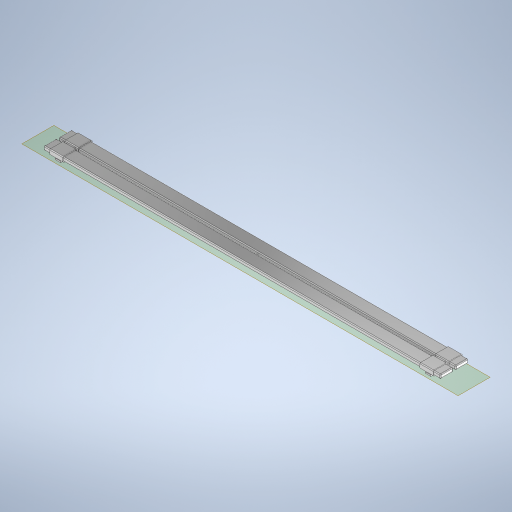
# Autodesk Inventor part: slider
Saved by Autodesk Inventor 2023 (Build 270158000, 158)
## iProperties
Created: 2023-11-22
Part Number: slider
Material: Aluminum 6061
Document SubType Name: Modeling
Designer: Beatrice
Density: 2.7 g/cm^3
Appearance: Chrome - Polished
Author: Beatrice
Autodesk Inventor part; units mm, degrees
ref_plane "YZ Plane" through (0, 0, 0) normal (1, 0, 0) x (0, 1, 0)
sketch "Sketch1" plane through (0, 0, 0) normal (1, 0, 0) x (0, 1, 0)
  line L0 (-1.5, -4.5) -> (-11.85, -4.5) construction
  line L1 (-11.85, -4.5) -> (-11.85, 0.0128) construction
  line L2 (-11.85, 0.0128) -> (0, 0.0128) construction
  line L3 (0, 0.0128) -> (0, 0) construction
  line L4 (0, 0) -> (2, 0) construction
  line L5 (2, 0) -> (2, -26) construction
  line L6 (2, -26) -> (0, -26) construction
  line L7 (0, -26) -> (-11.85, -26) construction
  line L8 (-11.85, -26) -> (-11.85, -21) construction
  line L9 (-11.85, -21) -> (-1.5, -21) construction
  line L10 (-1.5, -21) -> (-1.5, -4.5) construction
  arc A0 (1.25, -12.7436) -> (1.25, -13.2436) centre (1.25, -12.9936) ccw construction
  arc A1 (1.25, -12.7436) -> (1.5, -12.4936) centre (1.25, -12.4936) ccw construction
  line L11 (1.5, -12.4936) -> (1.5, -7.7436) construction
  arc A2 (1.5, -7.7436) -> (1.25, -7.4936) centre (1.25, -7.7436) ccw construction
  line L12 (1.25, -7.4936) -> (-0.25, -7.4936) construction
  arc A3 (-0.25, -7.4936) -> (-0.5, -7.7436) centre (-0.25, -7.7436) ccw construction
  line L13 (-0.5, -7.7436) -> (-0.5, -12.4936) construction
  arc A4 (-0.5, -12.4936) -> (-0.25, -12.7436) centre (-0.25, -12.4936) ccw construction
  arc A5 (-0.25, -13.2436) -> (-0.25, -12.7436) centre (-0.25, -12.9936) ccw construction
  line L14 (-0.25, -13.2436) -> (-0.5, -13.2436) construction
  line L15 (-0.5, -13.2436) -> (-0.5, -18.2436) construction
  arc A6 (-0.5, -18.2436) -> (-0.25, -18.4936) centre (-0.25, -18.2436) ccw construction
  line L16 (-0.25, -18.4936) -> (1.25, -18.4936) construction
  arc A7 (1.25, -18.4936) -> (1.5, -18.2436) centre (1.25, -18.2436) ccw construction
  line L17 (1.5, -18.2436) -> (1.5, -13.4936) construction
  arc A8 (1.5, -13.4936) -> (1.25, -13.2436) centre (1.25, -13.4936) ccw construction
  line L18 (-16, -26) -> (-16, 0.0128) construction
  line L19 (-16, 0.0128) -> (-12, 0.0128) construction
  line L20 (-12, 0.0128) -> (-12, -4.5) construction
  line L21 (-12, -4.5) -> (-15, -4.5) construction
  line L22 (-15, -4.5) -> (-15, -21) construction
  line L23 (-15, -21) -> (-12, -21) construction
  line L24 (-12, -21) -> (-12, -26) construction
  line L25 (-12, -26) -> (-16, -26) construction
  line L26 (-1.5, -4.5) -> (-11.85, -4.5) construction
  line L27 (-11.85, -4.5) -> (-11.85, 0.0128) construction
  line L28 (-11.85, 0.0128) -> (0, 0.0128) construction
  line L29 (0, 0.0128) -> (0, 0) construction
  line L30 (0, 0) -> (2, 0) construction
  line L31 (2, 0) -> (2, -26) construction
  line L32 (2, -26) -> (0, -26) construction
  line L33 (0, -26) -> (-11.85, -26) construction
  line L34 (-11.85, -26) -> (-11.85, -21) construction
  line L35 (-11.85, -21) -> (-1.5, -21) construction
  line L36 (-1.5, -21) -> (-1.5, -4.5) construction
  arc A9 (1.25, -12.7436) -> (1.25, -13.2436) centre (1.25, -12.9936) ccw construction
  arc A10 (1.25, -12.7436) -> (1.5, -12.4936) centre (1.25, -12.4936) ccw construction
  line L37 (1.5, -12.4936) -> (1.5, -7.7436) construction
  arc A11 (1.5, -7.7436) -> (1.25, -7.4936) centre (1.25, -7.7436) ccw construction
  line L38 (1.25, -7.4936) -> (-0.25, -7.4936) construction
  arc A12 (-0.25, -7.4936) -> (-0.5, -7.7436) centre (-0.25, -7.7436) ccw construction
  line L39 (-0.5, -7.7436) -> (-0.5, -12.4936) construction
  arc A13 (-0.5, -12.4936) -> (-0.25, -12.7436) centre (-0.25, -12.4936) ccw construction
  arc A14 (-0.25, -13.2436) -> (-0.25, -12.7436) centre (-0.25, -12.9936) ccw construction
  line L40 (-0.25, -13.2436) -> (-0.5, -13.2436) construction
  line L41 (-0.5, -13.2436) -> (-0.5, -18.2436) construction
  arc A15 (-0.5, -18.2436) -> (-0.25, -18.4936) centre (-0.25, -18.2436) ccw construction
  line L42 (-0.25, -18.4936) -> (1.25, -18.4936) construction
  arc A16 (1.25, -18.4936) -> (1.5, -18.2436) centre (1.25, -18.2436) ccw construction
  line L43 (1.5, -18.2436) -> (1.5, -13.4936) construction
  arc A17 (1.5, -13.4936) -> (1.25, -13.2436) centre (1.25, -13.4936) ccw construction
  line L44 (-16, -26) -> (-16, 0.0128) construction
  line L45 (-16, 0.0128) -> (-12, 0.0128) construction
  line L46 (-12, 0.0128) -> (-12, -4.5) construction
  line L47 (-12, -4.5) -> (-15, -4.5) construction
  line L48 (-15, -4.5) -> (-15, -21) construction
  line L49 (-15, -21) -> (-12, -21) construction
  line L50 (-12, -21) -> (-12, -26) construction
  line L51 (-12, -26) -> (-16, -26) construction
  line L52 (2.5, -25.5) -> (2.5, -0.5) construction
  circle A18 centre (2.5, 0.0128) radius 4.5 construction
  arc A19 (-10.2564, 1.2628) -> (-10.7564, 1.2628) centre (-10.5064, 1.2628) ccw construction
  arc A20 (-10.2564, 1.2628) -> (-10.7564, 1.2628) centre (-10.5064, 1.2628) ccw construction
  arc A21 (-10.0064, 3.0128) -> (-10.2564, 2.7628) centre (-10.0064, 2.7628) ccw construction
  line L53 (-18.5128, 14.3628) -> (-18.5128, 4.0128) construction
  line L54 (-18.5128, 4.0128) -> (-2.0128, 4.0128) construction
  line L55 (-18.5128, 4.0128) -> (-2.0128, 4.0128) construction
  line L56 (-23.5128, 2.5128) -> (-23.5128, 14.3628) construction
  line L57 (-2.0128, 17.5128) -> (-18.5128, 17.5128) construction
  line L58 (-2.0128, 17.5128) -> (-18.5128, 17.5128) construction
  line L59 (-23.0128, 0.0128) -> (1.9872, 0.0128) construction
  line L60 (-23.5128, 18.5128) -> (2.5, 18.5128) construction
  line L61 (-23.5128, 18.5128) -> (2.5, 18.5128) construction
  line L62 (2.4872, 0.5128) -> (-23.5128, 0.5128) construction
  line L63 (2.4872, 0.5128) -> (-23.5128, 0.5128) construction
  arc A22 (-10.2564, 1.2628) -> (-10.0064, 1.0128) centre (-10.0064, 1.2628) ccw construction
  line L64 (-10.0064, 1.0128) -> (-5.2564, 1.0128) construction
  arc A23 (-5.2564, 1.0128) -> (-5.0064, 1.2628) centre (-5.2564, 1.2628) ccw construction
  line L65 (-23.5128, 14.3628) -> (-18.5128, 14.3628) construction
  line L66 (-2.0128, 4.0128) -> (-2.0128, 14.3628) construction
  line L67 (-2.0128, 14.3628) -> (2.5, 14.3628) construction
  line L68 (2.5, 14.3628) -> (2.5, 2.5128) construction
  line L69 (-23.5128, 0.5128) -> (-23.5128, 2.5128) construction
  arc A24 (-10.7564, 2.7628) -> (-10.2564, 2.7628) centre (-10.5064, 2.7628) ccw construction
  arc A25 (-10.7564, 2.7628) -> (-10.2564, 2.7628) centre (-10.5064, 2.7628) ccw construction
  line L70 (-5.2564, 3.0128) -> (-10.0064, 3.0128) construction
  arc A26 (-5.0064, 2.7628) -> (-5.2564, 3.0128) centre (-5.2564, 2.7628) ccw construction
  line L71 (-10.7564, 2.7628) -> (-10.7564, 3.0128) construction
  line L72 (-10.7564, 2.7628) -> (-10.7564, 3.0128) construction
  arc A27 (-11.0064, 1.0128) -> (-10.7564, 1.2628) centre (-11.0064, 1.2628) ccw construction
  line L73 (-15.7564, 1.0128) -> (-11.0064, 1.0128) construction
  line L74 (-15.7564, 1.0128) -> (-11.0064, 1.0128) construction
  line L75 (-10.7564, 3.0128) -> (-15.7564, 3.0128) construction
  line L76 (-10.7564, 3.0128) -> (-15.7564, 3.0128) construction
  arc A28 (-15.7564, 3.0128) -> (-16.0064, 2.7628) centre (-15.7564, 2.7628) ccw construction
  arc A29 (-15.7564, 3.0128) -> (-16.0064, 2.7628) centre (-15.7564, 2.7628) ccw construction
  arc A30 (-11.0064, 1.0128) -> (-10.7564, 1.2628) centre (-11.0064, 1.2628) ccw construction
  line L77 (2.5, 2.5128) -> (2.4872, 2.5128) construction
  line L78 (2.4872, 2.5128) -> (2.4872, 0.5128) construction
  line L79 (-5.0064, 1.2628) -> (-5.0064, 2.7628) construction
  line L80 (-2.0128, 4.0128) -> (-2.0128, 14.3628) construction
  line L81 (2.5, 14.3628) -> (2.5, 2.5128) construction
  arc A31 (-16.0064, 1.2628) -> (-15.7564, 1.0128) centre (-15.7564, 1.2628) ccw construction
  arc A32 (-16.0064, 1.2628) -> (-15.7564, 1.0128) centre (-15.7564, 1.2628) ccw construction
  line L82 (-16.0064, 2.7628) -> (-16.0064, 1.2628) construction
  line L83 (-16.0064, 2.7628) -> (-16.0064, 1.2628) construction
  line L84 (-2.0128, 14.5128) -> (-2.0128, 17.5128) construction
  line L85 (-2.0128, 14.3628) -> (2.5, 14.3628) construction
  line L86 (2.5, 14.5128) -> (-2.0128, 14.5128) construction
  line L87 (2.5, 18.5128) -> (2.5, 14.5128) construction
  arc A33 (-10.2564, 1.2628) -> (-10.0064, 1.0128) centre (-10.0064, 1.2628) ccw construction
  line L88 (-5.2564, 3.0128) -> (-10.0064, 3.0128) construction
  arc A34 (-5.0064, 2.7628) -> (-5.2564, 3.0128) centre (-5.2564, 2.7628) ccw construction
  line L89 (-10.0064, 1.0128) -> (-5.2564, 1.0128) construction
  arc A35 (-5.2564, 1.0128) -> (-5.0064, 1.2628) centre (-5.2564, 1.2628) ccw construction
  arc A36 (-10.0064, 3.0128) -> (-10.2564, 2.7628) centre (-10.0064, 2.7628) ccw construction
  line L90 (2.5, 2.5128) -> (2.4872, 2.5128) construction
  line L91 (2.4872, 2.5128) -> (2.4872, 0.5128) construction
  line L92 (-5.0064, 1.2628) -> (-5.0064, 2.7628) construction
  circle A37 centre (2.5, 0.0128) radius 4.5 construction
  line L93 (-18.5128, 17.5128) -> (-18.5128, 14.5128) construction
  line L94 (-18.5128, 17.5128) -> (-18.5128, 14.5128) construction
  line L95 (-23.5128, 0.5128) -> (-23.5128, 2.5128) construction
  line L96 (-23.5128, 2.5128) -> (-23.5128, 14.3628) construction
  line L97 (-23.5128, 14.3628) -> (-18.5128, 14.3628) construction
  line L98 (-18.5128, 14.5128) -> (-23.5128, 14.5128) construction
  line L99 (-18.5128, 14.5128) -> (-23.5128, 14.5128) construction
  line L100 (-23.5128, 14.5128) -> (-23.5128, 18.5128) construction
  line L101 (-23.5128, 14.5128) -> (-23.5128, 18.5128) construction
  line L102 (-18.5128, 14.3628) -> (-18.5128, 4.0128) construction
  line L103 (2.5, 14.5128) -> (-2.0128, 14.5128) construction
  line L104 (2.5, 18.5128) -> (2.5, 14.5128) construction
  line L105 (-2.0128, 14.5128) -> (-2.0128, 17.5128) construction
  line L106 (-15.7564, 1.2628) -> (-11.0064, 1.2628)
  line L107 (-11.0064, 1.2628) -> (-11.0064, 2.7628)
  line L108 (-11.0064, 2.7628) -> (-15.7564, 2.7628)
  line L109 (-15.7564, 2.7628) -> (-15.7564, 1.2628)
  line L110 (-10.0064, 1.2628) -> (-5.2564, 1.2628)
  line L111 (-5.2564, 1.2628) -> (-5.2564, 2.7628)
  line L112 (-5.2564, 2.7628) -> (-10.0064, 2.7628)
  line L113 (-10.0064, 2.7628) -> (-10.0064, 1.2628)
  line L114 (-16.0064, 3.0128) -> (-10.7564, 3.0128)
  line L115 (-10.7564, 3.0128) -> (-10.7564, 1.0128)
  line L116 (-10.7564, 1.0128) -> (-16.0064, 1.0128)
  line L117 (-16.0064, 1.0128) -> (-16.0064, 3.0128)
  line L118 (-5.0064, 3.0128) -> (-10.2564, 3.0128)
  line L119 (-10.2564, 3.0128) -> (-10.2564, 1.0128)
  line L120 (-10.2564, 1.0128) -> (-5.0064, 1.0128)
  line L121 (-5.0064, 1.0128) -> (-5.0064, 3.0128)
  line L122 (-10.7564, 2.7628) -> (-10.2564, 2.7628)
  line L123 (-10.2564, 2.7628) -> (-10.2564, 1.2628)
  line L124 (-10.2564, 1.2628) -> (-10.7564, 1.2628)
  line L125 (-10.7564, 1.2628) -> (-10.7564, 2.7628)
  line L126 (-13.3814, 1.0128) -> (-14.8814, 1.0128)
  line L127 (-14.8814, 1.0128) -> (-14.8814, 0.0128)
  line L128 (-14.8814, 0.0128) -> (-13.3814, 0.0128)
  line L129 (-13.3814, 0.0128) -> (-13.3814, 1.0128)
  line L130 (-7.6314, 1.0128) -> (-6.1314, 1.0128)
  line L131 (-6.1314, 1.0128) -> (-6.1314, 0.0128)
  line L132 (-6.1314, 0.0128) -> (-7.6314, 0.0128)
  line L133 (-7.6314, 0.0128) -> (-7.6314, 1.0128)
  line L134 (-15.4076, 0.5128) -> (-5.5595, 0.5128)
  line L135 (-5.5595, 0.5128) -> (-5.5595, 0.0128)
  line L136 (-5.5595, 0.0128) -> (-15.4076, 0.0128)
  line L137 (-15.4076, 0.0128) -> (-15.4076, 0.5128)
  line L138 (-10.7564, -0.2137) -> (-10.7564, 0.8155) construction
  line L139 (-10.2564, 0.8155) -> (-10.2564, -0.2137) construction
  line L140 (-10.7564, 0.5128) -> (-10.2564, 0.5128)
  line L141 (-10.2564, 0.5128) -> (-10.2564, 0.4027)
  line L142 (-10.2564, 0.4027) -> (-10.7564, 0.4027)
  line L143 (-10.7564, 0.4027) -> (-10.7564, 0.5128)
  line L144 (-10.7564, 0.0128) -> (-10.2564, 0.0128)
  line L145 (-10.2564, 0.0128) -> (-10.2564, 0.1128)
  line L146 (-10.2564, 0.1128) -> (-10.7564, 0.1128)
  line L147 (-10.7564, 0.1128) -> (-10.7564, 0.0128)
  point P0 (-15, -12.9936)
  point P1 (-10.5064, 17.5128)
  point P2 (-13.3814, 0.5128)
  point P3 (-14.8814, 0.5128)
  point P4 (-14.8814, 0.0128)
  point P5 (-6.1314, 0.0128)
  point P6 (-6.1314, 0.5128)
  point P7 (-7.6314, 0.5128)
  dimension "d2" = 270
  dimension "d4" = 1.5
  dimension "d5" = 1.5
  dimension "d6" = 0.1
  constraints: 296 end point, 72 point on circle, 38 centre point, 20 parallel, 14 point on line, 11 perpendicular, 10 horizontal, 2 midpoint, 1 coincident, 1 vertical, 129 other
  measures "d4" distance of L128.end L127.end
  measures "d5" distance of L131.end L132.end
  measures "d6" distance of L145.end L144.end
extrude "Extrusion1" add sketch "Sketch1" along normal mid plane 2 contours L116 L129 L134 L127 | L134 L129 L128 L127 | L127 L136 L137 L134 | L134 L143 L142 L141 L133 L136 L145 L146 L147 L129 | L120 L131 L134 L133 | L134 L131 L132 L133 | L134 L135 L136 L131
extrude "Extrusion2" add sketch "Sketch1" along normal blind 5 and the other way blind 70 contours L109 L108 L107 L106 | L113 L112 L111 L110
fillet "Fillet1" radius 0.3 16 edges at (-32.5, -15.7564, 2.7628) (-32.5, -15.7564, 1.2628) (-32.5, -11.0064, 2.7628) (-32.5, -10.0064, 2.7628) (-32.5, -10.0064, 1.2628) (-32.5, -11.0064, 1.2628) (-32.5, -5.2564, 1.2628) (-32.5, -5.2564, 2.7628) (5, -13.3814, 2.7628) (5, -15.7564, 2.0128) (5, -13.3814, 1.2628) (5, -11.0064, 2.0128) (5, -10.0064, 2.0128) (5, -7.6314, 2.7628) (5, -7.6314, 1.2628) (5, -5.2564, 2.0128)
extrude "Extrusion3" add sketch "Sketch1" along normal mid plane 5 contours L114 L115 L116 L117 | L119 L118 L121 L120
extrude "Extrusion4" add sketch "Sketch1" along normal mid plane 3 contours L122 L119 L124 L115
fillet "Fillet2" radius 0.2 8 edges at (0, -15.7564, 2.7628) (0, -15.7564, 1.2628) (0, -11.0064, 2.7628) (0, -11.0064, 1.2628) (0, -10.0064, 1.2628) (0, -5.2564, 1.2628) (0, -5.2564, 2.7628) (0, -10.0064, 2.7628)
chamfer "Chamfer1" distance 0.3 angle 45 8 edges at (0, -16.0064, 3.0128) (0, -16.0064, 1.0128) (0, -10.7564, 3.0128) (0, -10.2564, 3.0128) (0, -5.0064, 3.0128) (0, -10.2564, 1.0128) (0, -10.7564, 1.0128) (0, -5.0064, 1.0128)
fillet "Fillet3" radius 0.2 8 edges at (1, -14.1314, 1.0128) (1, -6.8814, 1.0128) (0, -14.8814, 1.0128) (0, -7.6314, 1.0128) (0, -13.3814, 1.0128) (0, -6.1314, 1.0128) (-1, -14.1314, 1.0128) (-1, -6.8814, 1.0128)
ref_plane "Work Plane1" through (-70, 0, 0) normal (-1, 0, 0) x (0, 0, 1)
mirror "Mirror1" about plane through (-70, 0, 0) normal (-1, 0, 0) of "Extrusion1", "Extrusion2", "Fillet1", "Extrusion3", "Extrusion4", "Fillet2", "Chamfer1", "Fillet3"
ref_plane "Work Plane2" through (-2.5, -10.5064, 1.3128) normal (0, 1, 0) x (1, 0, 0)
ref_plane "Work Plane3" through (1, -10.7564, 0.0128) normal (0, 0, -1) x (-1, 0, 0)
body "Solid1"
